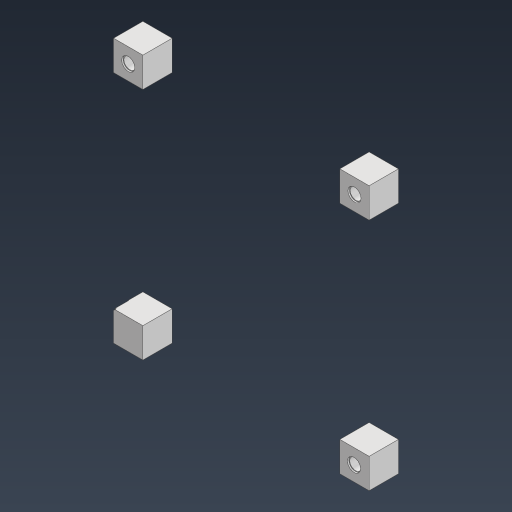
# Autodesk Inventor part: bms_hold_2
Saved by Autodesk Inventor 2023 (Build 270158000, 158)
## iProperties
Created: 2026-01-23
Part Number: bms_hold_2
Material: Generic
Document SubType Name: Modeling
Designer: szymo
Density: 1 g/cm^3
Appearance: Default
Author: szymo
Autodesk Inventor part; units mm, degrees
ref_plane "YZ Plane" through (0, 0, 0) normal (1, 0, 0) x (0, 1, 0)
ref_plane "XZ Plane" through (0, 0, 0) normal (0, 1, 0) x (-1, 0, 0)
ref_plane "XY Plane" through (0, 0, 0) normal (0, 0, 1) x (1, 0, 0)
sketch "Sketch1" plane through (0, 0, 0) normal (0, 0, 1) x (1, 0, 0)
  circle A0 centre (-5.1878, 0) radius 1.8 projected
  line L0 (-10.075, 5.075) -> (10.075, 5.075) projected
  line L1 (-10.075, -5.075) -> (-10.075, 5.075) projected
  line L2 (10.075, -5.075) -> (-10.075, -5.075) projected
  line L3 (10.075, 5.075) -> (10.075, -5.075) projected
  circle A1 centre (71.9239, 0) radius 1.8 projected
  line L4 (56.925, -5.075) -> (56.925, 5.075) projected
  line L5 (77.075, -5.075) -> (56.925, -5.075) projected
  line L6 (77.075, 5.075) -> (77.075, -5.075) projected
  line L7 (56.925, 5.075) -> (77.075, 5.075) projected
  circle A2 centre (72.075, -79.9) radius 1.8 projected
  line L8 (77.075, -84.975) -> (56.925, -84.975) projected
  line L9 (77.075, -74.825) -> (77.075, -84.975) projected
  line L10 (56.925, -74.825) -> (77.075, -74.825) projected
  line L11 (56.925, -84.975) -> (56.925, -74.825) projected
  circle A3 centre (-4.8097, -79.7917) radius 1.8 projected
  line L12 (-10.075, -74.825) -> (10.075, -74.825) projected
  line L13 (-10.075, -84.975) -> (-10.075, -74.825) projected
  line L14 (10.075, -84.975) -> (-10.075, -84.975) projected
  line L15 (10.075, -74.825) -> (10.075, -84.975) projected
  line L16 (-10.075, 5.075) -> (-0.075, 5.075)
  line L17 (-0.075, 5.075) -> (-0.075, -5.075)
  line L18 (-0.075, -5.075) -> (-10.075, -5.075)
  line L19 (-10.075, -5.075) -> (-10.075, 5.075)
  line L20 (-10.075, -74.825) -> (-0.075, -74.825)
  line L21 (-0.075, -74.825) -> (-0.075, -84.975)
  line L22 (-0.075, -84.975) -> (-10.075, -84.975)
  line L23 (-10.075, -84.975) -> (-10.075, -74.825)
  line L24 (77.075, -74.825) -> (67.075, -74.825)
  line L25 (67.075, -74.825) -> (67.075, -84.975)
  line L26 (67.075, -84.975) -> (77.075, -84.975)
  line L27 (77.075, -84.975) -> (77.075, -74.825)
  line L28 (77.075, -5.075) -> (67.075, -5.075)
  line L29 (67.075, -5.075) -> (67.075, 5.075)
  line L30 (67.075, 5.075) -> (77.075, 5.075)
  line L31 (77.075, 5.075) -> (77.075, -5.075)
  circle A4 centre (5, 0) radius 2.575 projected
  circle A5 centre (5, -79.9) radius 2.575 projected
  circle A6 centre (62, -79.9) radius 2.575 projected
  circle A7 centre (62, 0) radius 2.575 projected
  point P0 (0, 0)
  point P1 (-0.075, -74.825)
  point P2 (67.075, -74.825)
  point P3 (67.075, -5.075)
  point P4 (-0.075, 5.075)
  point P5 (7.4746, 0.7121)
  point P6 (2.5254, 0.7121)
  point P7 (-0.075, 5.075)
  point P8 (64.4746, -79.1879)
  point P9 (59.5254, -79.1879)
  point P10 (7.4746, -79.1879)
  point P11 (2.5254, -79.1879)
  point P12 (-0.075, -74.825)
  point P13 (64.4746, 0.7121)
  point P14 (59.5254, 0.7121)
  dimension "d0" = 10
  dimension "d1" = 10
  dimension "d2" = 10
  dimension "d3" = 10
  constraints: 32 end point, 8 parallel, 4 horizontal, 4 perpendicular, 4 point on line
  measures "d0" distance of L17.end L18.end
  measures "d1" distance of L21.end L22.end
  measures "d2" distance of L26.end L25.end
  measures "d3" distance of L29.end L30.end
extrude "Extrusion1" add sketch "Sketch1" along normal blind 10 contours A0 | L0 L17 L2 L1 | A1 | L29 L7 L6 L5 | A2 | L8 L25 L10 L9 | A3 | L12 L21 L14 L13
sketch "Sketch2" plane through (0, 0, 10) normal (0, 0, 1) x (1, 0, 0)
  line L0 (-0.075, 5.075) -> (-10.075, 5.075) projected
  line L1 (-10.075, -5.075) -> (-0.075, -5.075) projected
  line L2 (67.075, -5.075) -> (77.075, -5.075) projected
  line L3 (77.075, -5.075) -> (77.075, 5.075) projected
  line L4 (77.075, 5.075) -> (67.075, 5.075) projected
  line L5 (67.075, 5.075) -> (67.075, -5.075) projected
  line L6 (67.075, -84.975) -> (77.075, -84.975) projected
  line L7 (77.075, -84.975) -> (77.075, -74.825) projected
  line L8 (77.075, -74.825) -> (67.075, -74.825) projected
  line L9 (67.075, -74.825) -> (67.075, -84.975) projected
  line L10 (-0.075, -74.825) -> (-10.075, -74.825) projected
  line L11 (-10.075, -84.975) -> (-0.075, -84.975) projected
  line L12 (-10.075, 5.075) -> (-0.075, 5.075)
  line L13 (-10.075, -5.075) -> (-0.075, 5.075)
  line L14 (77.075, 5.075) -> (67.075, 5.075) projected
  line L15 (67.075, 5.075) -> (77.075, -5.075)
  line L16 (77.075, -74.825) -> (66.7728, -84.975)
  line L17 (-12.7422, -72.1178) -> (-10.075, -74.825)
  line L18 (-10.075, -74.825) -> (-10.075, -84.975) projected
  line L19 (-10.075, 5.075) -> (-10.075, -5.075) projected
  line L20 (-0.075, -84.975) -> (-0.075, -74.825) projected
  line L21 (-0.075, -5.075) -> (-0.075, 5.075) projected
  point P0 (0, 0)
  point P1 (-5.075, 0)
  point P2 (72.075, 0)
  point P3 (71.9239, -79.9)
  point P4 (-11.4086, -73.4714)
  constraints: 10 end point, 4 midpoint, 2 perpendicular, 1 point on line
hole "Hole1" at (72.075, 0, 10) at (71.9239, -79.9, 10) at (-11.4086, -73.4714, 10) at (-5.075, 0, 10) direction (0, 0, -1) diameter 4 depth 5 counterbore diameter 4.5 counterbore depth 0.5
sketch "Sketch3" plane through (0, 0, 0) normal (0, 0, -1) x (-1, 0, 0)
  circle A0 centre (-71.9239, 0) radius 1.8 projected
  circle A1 centre (5.1878, 0) radius 1.8 projected
  circle A2 centre (4.8097, -79.7917) radius 1.8 projected
  circle A3 centre (-72.075, -79.9) radius 1.8 projected
  circle A4 centre (-72.075, 0) radius 2 projected
  circle A5 centre (5.075, 0) radius 2.25 projected
  circle A6 centre (-71.9239, -79.9) radius 2 projected
  point P0 (0, 0)
  point P1 (9.9362, -74.825)
  point P2 (10.075, -74.9619)
  constraints: 4 coincident
hole "Hole2" at (72.075, 0, 0) at (-5.075, 0, 0) at (71.9239, -79.9, 0) at (-4.8097, -79.7917, 0) direction (0, 0, 1) diameter 4 depth 5 counterbore diameter 4.5 counterbore depth 0.5
body "Solid1"
